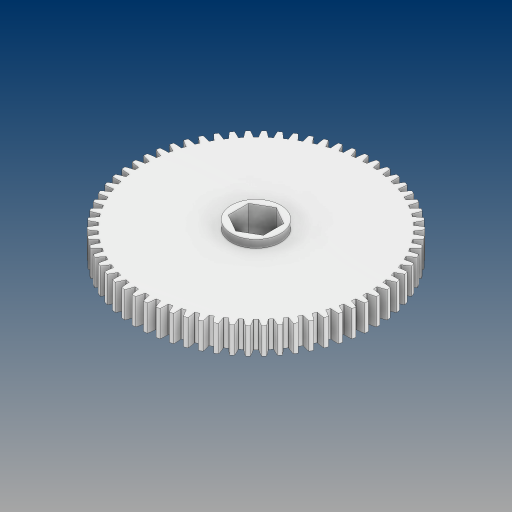
# Autodesk Inventor part: SHOT_1_004_66TGear-24TPulley
Saved by Autodesk Inventor 2024.3 (Build 283343000, 343)
## iProperties
Created: 2024-08-09
Part Number: SHOT_1_004_66TGear-24TPulley
Material: ABS Plastic
Document SubType Name: Modeling
Designer: Kenji
Density: 1.06 g/cm^3
Appearance: Smooth - White
Author: Kenji
Autodesk Inventor part; units mm, degrees
(part 1 of 3)
ref_plane "YZ Plane" through (0, 0, 0) normal (1, 0, 0) x (0, 1, 0)
ref_plane "XZ Plane" through (0, 0, 0) normal (0, 1, 0) x (-1, 0, 0)
ref_plane "XY Plane" through (0, 0, 0) normal (0, 0, 1) x (1, 0, 0)
sketch "Sketch1" plane through (0, 0, 0) normal (0, 1, 0) x (-1, 0, 0)
  circle A0 centre (0, 0) radius 41.91 construction
  line L0 (0, 0) -> (41.91, 0) construction
  line L1 (0, 0) -> (39.2827, 10.1592) construction
  line L2 (39.2827, 10.1592) -> (41.91, 0) construction
  arc A1 (39.2827, 10.1592) -> (37.9956, 14.2362) centre (0, 0) ccw construction
  arc A2 (40.5744, -0.225) -> (39.2827, 10.1592) centre (0, 0) ccw construction
  circle A3 centre (0, 0) radius 43.18
  line L3 (40.3225, 15.447) -> (40.3225, -15.447) construction
  line L4 (40.5744, -0.225) -> (41.91, 0) construction
  line L5 (40.5744, -0.225) -> (40.3225, -0.2901) construction
  line L6 (41.4814, 11.992) -> (38.8764, -18.7919) construction
  line L7 (40.5744, -0.225) -> (40.4457, -0.2469) construction
  line L8 (40.4457, -0.2469) -> (40.3225, -0.2901) construction
  line L9 (41.6879, 11.253) -> (38.5364, -19.4798) construction
  line L10 (40.5744, -0.225) -> (40.5099, -0.2348) construction
  line L11 (40.5099, -0.2348) -> (40.4457, -0.2469) construction
  line L12 (41.1912, 12.9537) -> (39.303, -17.8825) construction
  line L13 (40.5744, -0.225) -> (40.382, -0.2624) construction
  line L14 (40.4457, -0.2469) -> (40.382, -0.2624) construction
  line L15 (40.382, -0.2624) -> (40.3225, -0.2901) construction
  line L16 (37.9956, 14.2362) -> (43.1781, 0.4045) construction
  arc A4 (40.3121, -0.9596) -> (40.3225, -0.2901) centre (0, 0) ccw
  line L17 (40.3121, -0.9596) -> (0, 0) construction
  arc A5 (43.1678, -1.0276) -> (43.1781, 0.4045) centre (0, 0) ccw construction
  line L18 (43.1678, -1.0276) -> (40.3121, -0.9596) construction
  arc A6 (43.11, -2.4585) -> (43.1678, -1.0276) centre (0, 0) ccw construction
  arc A7 (40.2906, -1.6288) -> (40.3121, -0.9596) centre (0, 0) ccw
  line L19 (43.1781, 0.4045) -> (41.91, 0) construction
  line L20 (41.91, 0) -> (40.5744, -0.225) construction
  spline S0 degree 2 poles (43.1781, 0.4045) (41.91, 0) (40.5744, -0.225) knots 1 1 1 2 2 2
  line L21 (40.5744, -0.225) -> (40.5099, -0.2348) construction
  line L22 (40.5099, -0.2348) -> (40.4457, -0.2469) construction
  line L23 (40.4457, -0.2469) -> (40.382, -0.2624) construction
  line L24 (40.382, -0.2624) -> (40.3225, -0.2901) construction
  spline S1 degree 4 poles (40.5744, -0.225) (40.5099, -0.2348) (40.4457, -0.2469) (40.382, -0.2624) (40.3225, -0.2901) knots 1 1 1 1 1 2 2 2 2 2
  line L25 (43.11, -2.4585) -> (41.8625, -1.9942) construction
  line L26 (41.8625, -1.9942) -> (40.5392, -1.7059) construction
  spline S2 degree 2 poles (43.11, -2.4585) (41.8625, -1.9942) (40.5392, -1.7059) knots 1 1 1 2 2 2
  line L27 (40.5392, -1.7059) -> (40.4752, -1.693) construction
  line L28 (40.4752, -1.693) -> (40.4117, -1.6779) construction
  line L29 (40.4117, -1.6779) -> (40.3487, -1.6594) construction
  line L30 (40.3487, -1.6594) -> (40.2906, -1.6288) construction
  spline S3 degree 4 poles (40.5392, -1.7059) (40.4752, -1.693) (40.4117, -1.6779) (40.3487, -1.6594) (40.2906, -1.6288) knots 1 1 1 1 1 2 2 2 2 2
  line L31 (42.9441, 4.507) -> (41.7202, 3.9838) construction
  spline S4 degree 2 poles (42.9441, 4.507) (41.7202, 3.9838) (40.4121, 3.6329) knots 1 1 1 2 2 2
  line L32 (41.7202, 3.9838) -> (40.4121, 3.6329) construction
  spline S5 degree 2 poles (43.1484, 1.6505) (41.8625, 1.9942) (40.5178, 2.1553) knots 1 1 1 2 2 2
  line L33 (43.1484, 1.6505) -> (41.8625, 1.9942) construction
  line L34 (41.8625, 1.9942) -> (40.5178, 2.1553) construction
  line L35 (40.4528, 2.1621) -> (40.3882, 2.1711) construction
  spline S6 degree 4 poles (40.5178, 2.1553) (40.4528, 2.1621) (40.3882, 2.1711) (40.3237, 2.1835) (40.263, 2.2084) knots 1 1 1 1 1 2 2 2 2 2
  line L36 (40.5178, 2.1553) -> (40.4528, 2.1621) construction
  line L37 (40.3882, 2.1711) -> (40.3237, 2.1835) construction
  line L38 (40.3237, 2.1835) -> (40.263, 2.2084) construction
  arc A8 (40.263, 2.2084) -> (40.2208, 2.8766) centre (0, 0) ccw
  arc A9 (40.2208, 2.8766) -> (40.1675, 3.5441) centre (0, 0) ccw
  spline S7 degree 4 poles (40.4121, 3.6329) (40.3488, 3.617) (40.286, 3.5988) (40.224, 3.5774) (40.1675, 3.5441) knots 1 1 1 1 1 2 2 2 2 2
  line L39 (40.4121, 3.6329) -> (40.3488, 3.617) construction
  line L40 (40.3488, 3.617) -> (40.286, 3.5988) construction
  line L41 (40.286, 3.5988) -> (40.224, 3.5774) construction
  line L42 (40.224, 3.5774) -> (40.1675, 3.5441) construction
  line L43 (42.3213, 8.5687) -> (41.1526, 7.9315) construction
  spline S8 degree 2 poles (42.3213, 8.5687) (41.1526, 7.9315) (39.8838, 7.4578) knots 1 1 1 2 2 2
  line L44 (41.1526, 7.9315) -> (39.8838, 7.4578) construction
  spline S9 degree 2 poles (42.7962, 5.7445) (41.4834, 5.9644) (40.1294, 5.997) knots 1 1 1 2 2 2
  line L45 (42.7962, 5.7445) -> (41.4834, 5.9644) construction
  line L46 (41.4834, 5.9644) -> (40.1294, 5.997) construction
  line L47 (40.0641, 5.9976) -> (39.9989, 6.0004) construction
  spline S10 degree 4 poles (40.1294, 5.997) (40.0641, 5.9976) (39.9989, 6.0004) (39.9336, 6.0067) (39.8708, 6.0257) knots 1 1 1 1 1 2 2 2 2 2
  line L48 (40.1294, 5.997) -> (40.0641, 5.9976) construction
  line L49 (39.9989, 6.0004) -> (39.9336, 6.0067) construction
  line L50 (39.9336, 6.0067) -> (39.8708, 6.0257) construction
  arc A10 (39.8708, 6.0257) -> (39.7652, 6.6869) centre (0, 0) ccw
  arc A11 (39.7652, 6.6869) -> (39.6487, 7.3462) centre (0, 0) ccw
  spline S11 degree 4 poles (39.8838, 7.4578) (39.8223, 7.436) (39.7615, 7.412) (39.7019, 7.3847) (39.6487, 7.3462) knots 1 1 1 1 1 2 2 2 2 2
  line L51 (39.8838, 7.4578) -> (39.8223, 7.436) construction
  line L52 (39.8223, 7.436) -> (39.7615, 7.412) construction
  line L53 (39.7615, 7.412) -> (39.7019, 7.3847) construction
  line L54 (39.7019, 7.3847) -> (39.6487, 7.3462) construction
  line L55 (41.3151, 12.5528) -> (40.2124, 11.8074) construction
  spline S12 degree 2 poles (41.3151, 12.5528) (40.2124, 11.8074) (38.9943, 11.2153) knots 1 1 1 2 2 2
  line L56 (40.2124, 11.8074) -> (38.9943, 11.2153) construction
  spline S13 degree 2 poles (42.0563, 9.7866) (40.7286, 9.8807) (39.3777, 9.7844) knots 1 1 1 2 2 2
  line L57 (42.0563, 9.7866) -> (40.7286, 9.8807) construction
  line L58 (40.7286, 9.8807) -> (39.3777, 9.7844) construction
  line L59 (39.3126, 9.7787) -> (39.2474, 9.7754) construction
  spline S14 degree 4 poles (39.3777, 9.7844) (39.3126, 9.7787) (39.2474, 9.7754) (39.1818, 9.7754) (39.1175, 9.7883) knots 1 1 1 1 1 2 2 2 2 2
  line L60 (39.3777, 9.7844) -> (39.3126, 9.7787) construction
  line L61 (39.2474, 9.7754) -> (39.1818, 9.7754) construction
  line L62 (39.1818, 9.7754) -> (39.1175, 9.7883) construction
  arc A12 (39.1175, 9.7883) -> (38.9496, 10.4365) centre (0, 0) ccw
  arc A13 (38.9496, 10.4365) -> (38.7709, 11.0818) centre (0, 0) ccw
  spline S15 degree 4 poles (38.9943, 11.2153) (38.9351, 11.1877) (38.8769, 11.158) (38.8201, 11.1252) (38.7709, 11.0818) knots 1 1 1 1 1 2 2 2 2 2
  line L63 (38.9943, 11.2153) -> (38.9351, 11.1877) construction
  line L64 (38.9351, 11.1877) -> (38.8769, 11.158) construction
  line L65 (38.8769, 11.158) -> (38.8201, 11.1252) construction
  line L66 (38.8201, 11.1252) -> (38.7709, 11.0818) construction
  line L67 (39.9348, 16.4232) -> (38.9079, 15.5764) construction
  spline S16 degree 2 poles (39.9348, 16.4232) (38.9079, 15.5764) (37.7516, 14.8711) knots 1 1 1 2 2 2
  line L68 (38.9079, 15.5764) -> (37.7516, 14.8711) construction
  spline S17 degree 2 poles (40.9356, 13.7399) (39.605, 13.7074) (38.2693, 13.4832) knots 1 1 1 2 2 2
  line L69 (40.9356, 13.7399) -> (39.605, 13.7074) construction
  line L70 (39.605, 13.7074) -> (38.2693, 13.4832) construction
  line L71 (38.2051, 13.4714) -> (38.1405, 13.4618) construction
  spline S18 degree 4 poles (38.2693, 13.4832) (38.2051, 13.4714) (38.1405, 13.4618) (38.0752, 13.4556) (38.0099, 13.4624) knots 1 1 1 1 1 2 2 2 2 2
  line L72 (38.2693, 13.4832) -> (38.2051, 13.4714) construction
  line L73 (38.1405, 13.4618) -> (38.0752, 13.4556) construction
  line L74 (38.0752, 13.4556) -> (38.0099, 13.4624) construction
  arc A14 (38.0099, 13.4624) -> (37.7811, 14.0916) centre (0, 0) ccw
  arc A15 (37.7811, 14.0916) -> (37.5419, 14.717) centre (0, 0) ccw
  spline S19 degree 4 poles (37.7516, 14.8711) (37.6953, 14.838) (37.6403, 14.8029) (37.5868, 14.7649) (37.5419, 14.717) knots 1 1 1 1 1 2 2 2 2 2
  line L75 (37.7516, 14.8711) -> (37.6953, 14.838) construction
  line L76 (37.6953, 14.838) -> (37.6403, 14.8029) construction
  line L77 (37.6403, 14.8029) -> (37.5868, 14.7649) construction
  line L78 (37.5868, 14.7649) -> (37.5419, 14.717) construction
  line L79 (38.1929, 20.1449) -> (37.2511, 19.2043) construction
  spline S20 degree 2 poles (38.1929, 20.1449) (37.2511, 19.2043) (36.1671, 18.3923) knots 1 1 1 2 2 2
  line L80 (37.2511, 19.2043) -> (36.1671, 18.3923) construction
  spline S21 degree 2 poles (39.4442, 17.5689) (38.1227, 17.41) (36.8144, 17.0599) knots 1 1 1 2 2 2
  line L81 (39.4442, 17.5689) -> (38.1227, 17.41) construction
  line L82 (38.1227, 17.41) -> (36.8144, 17.0599) construction
  line L83 (36.7515, 17.042) -> (36.6882, 17.0263) construction
  spline S22 degree 4 poles (36.8144, 17.0599) (36.7515, 17.042) (36.6882, 17.0263) (36.6237, 17.0139) (36.5581, 17.0145) knots 1 1 1 1 1 2 2 2 2 2
  line L84 (36.8144, 17.0599) -> (36.7515, 17.042) construction
  line L85 (36.6882, 17.0263) -> (36.6237, 17.0139) construction
  line L86 (36.6237, 17.0139) -> (36.5581, 17.0145) construction
  arc A16 (36.5581, 17.0145) -> (36.2706, 17.6192) centre (0, 0) ccw
  arc A17 (36.2706, 17.6192) -> (35.973, 18.219) centre (0, 0) ccw
  spline S23 degree 4 poles (36.1671, 18.3923) (36.1142, 18.354) (36.0627, 18.3138) (36.0131, 18.2709) (35.973, 18.219) knots 1 1 1 1 1 2 2 2 2 2
  line L87 (36.1671, 18.3923) -> (36.1142, 18.354) construction
  line L88 (36.1142, 18.354) -> (36.0627, 18.3138) construction
  line L89 (36.0627, 18.3138) -> (36.0131, 18.2709) construction
  line L90 (36.0131, 18.2709) -> (35.973, 18.219) construction
  line L91 (36.1051, 23.6841) -> (35.2569, 22.6583) construction
  spline S24 degree 2 poles (36.1051, 23.6841) (35.2569, 22.6583) (34.255, 21.7469) knots 1 1 1 2 2 2
  line L92 (35.2569, 22.6583) -> (34.255, 21.7469) construction
  spline S25 degree 2 poles (37.5956, 21.2388) (36.2951, 20.955) (35.026, 20.4821) knots 1 1 1 2 2 2
  line L93 (37.5956, 21.2388) -> (36.2951, 20.955) construction
  line L94 (36.2951, 20.955) -> (35.026, 20.4821) construction
  line L95 (34.9652, 20.4583) -> (34.9036, 20.4367) construction
  spline S26 degree 4 poles (35.026, 20.4821) (34.9652, 20.4583) (34.9036, 20.4367) (34.8406, 20.4182) (34.7752, 20.4125) knots 1 1 1 1 1 2 2 2 2 2
  line L96 (35.026, 20.4821) -> (34.9652, 20.4583) construction
  line L97 (34.9036, 20.4367) -> (34.8406, 20.4182) construction
  line L98 (34.8406, 20.4182) -> (34.7752, 20.4125) construction
  arc A18 (34.7752, 20.4125) -> (34.4315, 20.9871) centre (0, 0) ccw
  arc A19 (34.4315, 20.9871) -> (34.0783, 21.5559) centre (0, 0) ccw
  spline S27 degree 4 poles (34.255, 21.7469) (34.206, 21.7038) (34.1586, 21.6589) (34.1133, 21.6114) (34.0783, 21.5559) knots 1 1 1 1 1 2 2 2 2 2
  line L99 (34.255, 21.7469) -> (34.206, 21.7038) construction
  line L100 (34.206, 21.7038) -> (34.1586, 21.6589) construction
  line L101 (34.1586, 21.6589) -> (34.1133, 21.6114) construction
  line L102 (34.1133, 21.6114) -> (34.0783, 21.5559) construction
  line L103 (33.6903, 27.0089) -> (32.9435, 25.907) construction
  spline S28 degree 2 poles (33.6903, 27.0089) (32.9435, 25.907) (32.0327, 24.9046) knots 1 1 1 2 2 2
  line L104 (32.9435, 25.907) -> (32.0327, 24.9046) construction
  spline S29 degree 2 poles (35.4065, 24.7163) (34.1389, 24.3102) (32.9205, 23.7188) knots 1 1 1 2 2 2
  line L105 (35.4065, 24.7163) -> (34.1389, 24.3102) construction
  line L106 (34.1389, 24.3102) -> (32.9205, 23.7188) construction
  line L107 (32.8622, 23.6893) -> (32.8029, 23.6619) construction
  spline S30 degree 4 poles (32.9205, 23.7188) (32.8622, 23.6893) (32.8029, 23.6619) (32.742, 23.6376) (32.6774, 23.6257) knots 1 1 1 1 1 2 2 2 2 2
  line L108 (32.9205, 23.7188) -> (32.8622, 23.6893) construction
  line L109 (32.8029, 23.6619) -> (32.742, 23.6376) construction
  line L110 (32.742, 23.6376) -> (32.6774, 23.6257) construction
  arc A20 (32.6774, 23.6257) -> (32.2807, 24.165) centre (0, 0) ccw
  arc A21 (32.2807, 24.165) -> (31.875, 24.6977) centre (0, 0) ccw
  spline S31 degree 4 poles (32.0327, 24.9046) (31.9881, 24.857) (31.9451, 24.8078) (31.9046, 24.7562) (31.875, 24.6977) knots 1 1 1 1 1 2 2 2 2 2
  line L111 (32.0327, 24.9046) -> (31.9881, 24.857) construction
  line L112 (31.9881, 24.857) -> (31.9451, 24.8078) construction
  line L113 (31.9451, 24.8078) -> (31.9046, 24.7562) construction
  line L114 (31.9046, 24.7562) -> (31.875, 24.6977) construction
  line L115 (30.9703, 30.089) -> (30.3317, 28.9212) construction
  spline S32 degree 2 poles (30.9703, 30.089) (30.3317, 28.9212) (29.5204, 27.8367) knots 1 1 1 2 2 2
  line L116 (30.3317, 28.9212) -> (29.5204, 27.8367) construction
  spline S33 degree 2 poles (32.8967, 27.97) (31.6735, 27.4452) (30.5168, 26.7406) knots 1 1 1 2 2 2
  line L117 (32.8967, 27.97) -> (31.6735, 27.4452) construction
  line L118 (31.6735, 27.4452) -> (30.5168, 26.7406) construction
  line L119 (30.4616, 26.7058) -> (30.4051, 26.6729) construction
  spline S34 degree 4 poles (30.5168, 26.7406) (30.4616, 26.7058) (30.4051, 26.6729) (30.3468, 26.6429) (30.2837, 26.6249) knots 1 1 1 1 1 2 2 2 2 2
  line L120 (30.5168, 26.7406) -> (30.4616, 26.7058) construction
  line L121 (30.4051, 26.6729) -> (30.3468, 26.6429) construction
  line L122 (30.3468, 26.6429) -> (30.2837, 26.6249) construction
  arc A22 (30.2837, 26.6249) -> (29.8375, 27.1241) centre (0, 0) ccw
  arc A23 (29.8375, 27.1241) -> (29.383, 27.6157) centre (0, 0) ccw
  spline S35 degree 4 poles (29.5204, 27.8367) (29.4804, 27.7851) (29.4423, 27.732) (29.4069, 27.6768) (29.383, 27.6157) knots 1 1 1 1 1 2 2 2 2 2
  line L123 (29.5204, 27.8367) -> (29.4804, 27.7851) construction
  line L124 (29.4804, 27.7851) -> (29.4423, 27.732) construction
  line L125 (29.4423, 27.732) -> (29.4069, 27.6768) construction
  line L126 (29.4069, 27.6768) -> (29.383, 27.6157) construction
  line L127 (27.97, 32.8967) -> (27.4452, 31.6735) construction
  spline S36 degree 2 poles (27.97, 32.8967) (27.4452, 31.6735) (26.7406, 30.5168) knots 1 1 1 2 2 2
  line L128 (27.4452, 31.6735) -> (26.7406, 30.5168) construction
  spline S37 degree 2 poles (30.089, 30.9703) (28.9212, 30.3317) (27.8367, 29.5204) knots 1 1 1 2 2 2
  line L129 (30.089, 30.9703) -> (28.9212, 30.3317) construction
  line L130 (28.9212, 30.3317) -> (27.8367, 29.5204) construction
  line L131 (27.7851, 29.4804) -> (27.732, 29.4423) construction
  spline S38 degree 4 poles (27.8367, 29.5204) (27.7851, 29.4804) (27.732, 29.4423) (27.6768, 29.4069) (27.6157, 29.383) knots 1 1 1 1 1 2 2 2 2 2
  line L132 (27.8367, 29.5204) -> (27.7851, 29.4804) construction
  line L133 (27.732, 29.4423) -> (27.6768, 29.4069) construction
  line L134 (27.6768, 29.4069) -> (27.6157, 29.383) construction
  arc A24 (27.6157, 29.383) -> (27.1241, 29.8375) centre (0, 0) ccw
  arc A25 (27.1241, 29.8375) -> (26.6249, 30.2837) centre (0, 0) ccw
  spline S39 degree 4 poles (26.7406, 30.5168) (26.7058, 30.4616) (26.6729, 30.4051) (26.6429, 30.3468) (26.6249, 30.2837) knots 1 1 1 1 1 2 2 2 2 2
  line L135 (26.7406, 30.5168) -> (26.7058, 30.4616) construction
  line L136 (26.7058, 30.4616) -> (26.6729, 30.4051) construction
  line L137 (26.6729, 30.4051) -> (26.6429, 30.3468) construction
  line L138 (26.6429, 30.3468) -> (26.6249, 30.2837) construction
  line L139 (24.7163, 35.4065) -> (24.3102, 34.1389) construction
  spline S40 degree 2 poles (24.7163, 35.4065) (24.3102, 34.1389) (23.7188, 32.9205) knots 1 1 1 2 2 2
  line L140 (24.3102, 34.1389) -> (23.7188, 32.9205) construction
  spline S41 degree 2 poles (27.0089, 33.6903) (25.907, 32.9435) (24.9046, 32.0327) knots 1 1 1 2 2 2
  line L141 (27.0089, 33.6903) -> (25.907, 32.9435) construction
  line L142 (25.907, 32.9435) -> (24.9046, 32.0327) construction
  line L143 (24.857, 31.9881) -> (24.8078, 31.9451) construction
  spline S42 degree 4 poles (24.9046, 32.0327) (24.857, 31.9881) (24.8078, 31.9451) (24.7562, 31.9046) (24.6977, 31.875) knots 1 1 1 1 1 2 2 2 2 2
  line L144 (24.9046, 32.0327) -> (24.857, 31.9881) construction
  line L145 (24.8078, 31.9451) -> (24.7562, 31.9046) construction
  line L146 (24.7562, 31.9046) -> (24.6977, 31.875) construction
  arc A26 (24.6977, 31.875) -> (24.165, 32.2807) centre (0, 0) ccw
  arc A27 (24.165, 32.2807) -> (23.6257, 32.6774) centre (0, 0) ccw
  spline S43 degree 4 poles (23.7188, 32.9205) (23.6893, 32.8622) (23.6619, 32.8029) (23.6376, 32.742) (23.6257, 32.6774) knots 1 1 1 1 1 2 2 2 2 2
  line L147 (23.7188, 32.9205) -> (23.6893, 32.8622) construction
  line L148 (23.6893, 32.8622) -> (23.6619, 32.8029) construction
  line L149 (23.6619, 32.8029) -> (23.6376, 32.742) construction
  line L150 (23.6376, 32.742) -> (23.6257, 32.6774) construction
  line L151 (21.2388, 37.5956) -> (20.955, 36.2951) construction
  spline S44 degree 2 poles (21.2388, 37.5956) (20.955, 36.2951) (20.4821, 35.026) knots 1 1 1 2 2 2
  line L152 (20.955, 36.2951) -> (20.4821, 35.026) construction
  spline S45 degree 2 poles (23.6841, 36.1051) (22.6583, 35.2569) (21.7469, 34.255) knots 1 1 1 2 2 2
  line L153 (23.6841, 36.1051) -> (22.6583, 35.2569) construction
  line L154 (22.6583, 35.2569) -> (21.7469, 34.255) construction
  line L155 (21.7038, 34.206) -> (21.6589, 34.1586) construction
  spline S46 degree 4 poles (21.7469, 34.255) (21.7038, 34.206) (21.6589, 34.1586) (21.6114, 34.1133) (21.5559, 34.0783) knots 1 1 1 1 1 2 2 2 2 2
  line L156 (21.7469, 34.255) -> (21.7038, 34.206) construction
  line L157 (21.6589, 34.1586) -> (21.6114, 34.1133) construction
  line L158 (21.6114, 34.1133) -> (21.5559, 34.0783) construction
  arc A28 (21.5559, 34.0783) -> (20.9871, 34.4315) centre (0, 0) ccw
  arc A29 (20.9871, 34.4315) -> (20.4125, 34.7752) centre (0, 0) ccw
  spline S47 degree 4 poles (20.4821, 35.026) (20.4583, 34.9652) (20.4367, 34.9036) (20.4182, 34.8406) (20.4125, 34.7752) knots 1 1 1 1 1 2 2 2 2 2
  line L159 (20.4821, 35.026) -> (20.4583, 34.9652) construction
  line L160 (20.4583, 34.9652) -> (20.4367, 34.9036) construction
  line L161 (20.4367, 34.9036) -> (20.4182, 34.8406) construction
  line L162 (20.4182, 34.8406) -> (20.4125, 34.7752) construction
  line L163 (17.5689, 39.4442) -> (17.41, 38.1227) construction
  spline S48 degree 2 poles (17.5689, 39.4442) (17.41, 38.1227) (17.0599, 36.8144) knots 1 1 1 2 2 2
  line L164 (17.41, 38.1227) -> (17.0599, 36.8144) construction
  spline S49 degree 2 poles (20.1449, 38.1929) (19.2043, 37.2511) (18.3923, 36.1671) knots 1 1 1 2 2 2
  line L165 (20.1449, 38.1929) -> (19.2043, 37.2511) construction
  line L166 (19.2043, 37.2511) -> (18.3923, 36.1671) construction
  line L167 (18.354, 36.1142) -> (18.3138, 36.0627) construction
  spline S50 degree 4 poles (18.3923, 36.1671) (18.354, 36.1142) (18.3138, 36.0627) (18.2709, 36.0131) (18.219, 35.973) knots 1 1 1 1 1 2 2 2 2 2
  line L168 (18.3923, 36.1671) -> (18.354, 36.1142) construction
  line L169 (18.3138, 36.0627) -> (18.2709, 36.0131) construction
  line L170 (18.2709, 36.0131) -> (18.219, 35.973) construction
  arc A30 (18.219, 35.973) -> (17.6192, 36.2706) centre (0, 0) ccw
  arc A31 (17.6192, 36.2706) -> (17.0145, 36.5581) centre (0, 0) ccw
  spline S51 degree 4 poles (17.0599, 36.8144) (17.042, 36.7515) (17.0263, 36.6882) (17.0139, 36.6237) (17.0145, 36.5581) knots 1 1 1 1 1 2 2 2 2 2
  line L171 (17.0599, 36.8144) -> (17.042, 36.7515) construction
  line L172 (17.042, 36.7515) -> (17.0263, 36.6882) construction
  line L173 (17.0263, 36.6882) -> (17.0139, 36.6237) construction
  line L174 (17.0139, 36.6237) -> (17.0145, 36.5581) construction
  line L175 (13.7399, 40.9356) -> (13.7074, 39.605) construction
  spline S52 degree 2 poles (13.7399, 40.9356) (13.7074, 39.605) (13.4832, 38.2693) knots 1 1 1 2 2 2
  line L176 (13.7074, 39.605) -> (13.4832, 38.2693) construction
  spline S53 degree 2 poles (16.4232, 39.9348) (15.5764, 38.9079) (14.8711, 37.7516) knots 1 1 1 2 2 2
  line L177 (16.4232, 39.9348) -> (15.5764, 38.9079) construction
  line L178 (15.5764, 38.9079) -> (14.8711, 37.7516) construction
  line L179 (14.838, 37.6953) -> (14.8029, 37.6403) construction
  spline S54 degree 4 poles (14.8711, 37.7516) (14.838, 37.6953) (14.8029, 37.6403) (14.7649, 37.5868) (14.717, 37.5419) knots 1 1 1 1 1 2 2 2 2 2
  line L180 (14.8711, 37.7516) -> (14.838, 37.6953) construction
  line L181 (14.8029, 37.6403) -> (14.7649, 37.5868) construction
  line L182 (14.7649, 37.5868) -> (14.717, 37.5419) construction
  arc A32 (14.717, 37.5419) -> (14.0916, 37.7811) centre (0, 0) ccw
  arc A33 (14.0916, 37.7811) -> (13.4624, 38.0099) centre (0, 0) ccw
  spline S55 degree 4 poles (13.4832, 38.2693) (13.4714, 38.2051) (13.4618, 38.1405) (13.4556, 38.0752) (13.4624, 38.0099) knots 1 1 1 1 1 2 2 2 2 2
  line L183 (13.4832, 38.2693) -> (13.4714, 38.2051) construction
  line L184 (13.4714, 38.2051) -> (13.4618, 38.1405) construction
  line L185 (13.4618, 38.1405) -> (13.4556, 38.0752) construction
  line L186 (13.4556, 38.0752) -> (13.4624, 38.0099) construction
  line L187 (9.7866, 42.0563) -> (9.8807, 40.7286) construction
  spline S56 degree 2 poles (9.7866, 42.0563) (9.8807, 40.7286) (9.7844, 39.3777) knots 1 1 1 2 2 2
  line L188 (9.8807, 40.7286) -> (9.7844, 39.3777) construction
  spline S57 degree 2 poles (12.5528, 41.3151) (11.8074, 40.2124) (11.2153, 38.9943) knots 1 1 1 2 2 2
  line L189 (12.5528, 41.3151) -> (11.8074, 40.2124) construction
  line L190 (11.8074, 40.2124) -> (11.2153, 38.9943) construction
  line L191 (11.1877, 38.9351) -> (11.158, 38.8769) construction
  spline S58 degree 4 poles (11.2153, 38.9943) (11.1877, 38.9351) (11.158, 38.8769) (11.1252, 38.8201) (11.0818, 38.7709) knots 1 1 1 1 1 2 2 2 2 2
  line L192 (11.2153, 38.9943) -> (11.1877, 38.9351) construction
  line L193 (11.158, 38.8769) -> (11.1252, 38.8201) construction
  line L194 (11.1252, 38.8201) -> (11.0818, 38.7709) construction
  arc A34 (11.0818, 38.7709) -> (10.4365, 38.9496) centre (0, 0) ccw
  arc A35 (10.4365, 38.9496) -> (9.7883, 39.1175) centre (0, 0) ccw
  spline S59 degree 4 poles (9.7844, 39.3777) (9.7787, 39.3126) (9.7754, 39.2474) (9.7754, 39.1818) (9.7883, 39.1175) knots 1 1 1 1 1 2 2 2 2 2
  line L195 (9.7844, 39.3777) -> (9.7787, 39.3126) construction
  line L196 (9.7787, 39.3126) -> (9.7754, 39.2474) construction
  line L197 (9.7754, 39.2474) -> (9.7754, 39.1818) construction
  line L198 (9.7754, 39.1818) -> (9.7883, 39.1175) construction
  line L199 (5.7445, 42.7962) -> (5.9644, 41.4834) construction
  spline S60 degree 2 poles (5.7445, 42.7962) (5.9644, 41.4834) (5.997, 40.1294) knots 1 1 1 2 2 2
  line L200 (5.9644, 41.4834) -> (5.997, 40.1294) construction
  spline S61 degree 2 poles (8.5687, 42.3213) (7.9315, 41.1526) (7.4578, 39.8838) knots 1 1 1 2 2 2
  line L201 (8.5687, 42.3213) -> (7.9315, 41.1526) construction
  line L202 (7.9315, 41.1526) -> (7.4578, 39.8838) construction
  line L203 (7.436, 39.8223) -> (7.412, 39.7615) construction
  spline S62 degree 4 poles (7.4578, 39.8838) (7.436, 39.8223) (7.412, 39.7615) (7.3847, 39.7019) (7.3462, 39.6487) knots 1 1 1 1 1 2 2 2 2 2
  line L204 (7.4578, 39.8838) -> (7.436, 39.8223) construction
  line L205 (7.412, 39.7615) -> (7.3847, 39.7019) construction
  line L206 (7.3847, 39.7019) -> (7.3462, 39.6487) construction
  arc A36 (7.3462, 39.6487) -> (6.6869, 39.7652) centre (0, 0) ccw
  arc A37 (6.6869, 39.7652) -> (6.0257, 39.8708) centre (0, 0) ccw
  spline S63 degree 4 poles (5.997, 40.1294) (5.9976, 40.0641) (6.0004, 39.9989) (6.0067, 39.9336) (6.0257, 39.8708) knots 1 1 1 1 1 2 2 2 2 2
  line L207 (5.997, 40.1294) -> (5.9976, 40.0641) construction
  line L208 (5.9976, 40.0641) -> (6.0004, 39.9989) construction
  line L209 (6.0004, 39.9989) -> (6.0067, 39.9336) construction
  line L210 (6.0067, 39.9336) -> (6.0257, 39.8708) construction
  line L211 (1.6505, 43.1484) -> (1.9942, 41.8625) construction
  spline S64 degree 2 poles (1.6505, 43.1484) (1.9942, 41.8625) (2.1553, 40.5178) knots 1 1 1 2 2 2
  line L212 (1.9942, 41.8625) -> (2.1553, 40.5178) construction
  spline S65 degree 2 poles (4.507, 42.9441) (3.9838, 41.7202) (3.6329, 40.4121) knots 1 1 1 2 2 2
  line L213 (4.507, 42.9441) -> (3.9838, 41.7202) construction
  line L214 (3.9838, 41.7202) -> (3.6329, 40.4121) construction
  line L215 (3.617, 40.3488) -> (3.5988, 40.286) construction
  spline S66 degree 4 poles (3.6329, 40.4121) (3.617, 40.3488) (3.5988, 40.286) (3.5774, 40.224) (3.5441, 40.1675) knots 1 1 1 1 1 2 2 2 2 2
  line L216 (3.6329, 40.4121) -> (3.617, 40.3488) construction
  line L217 (3.5988, 40.286) -> (3.5774, 40.224) construction
  line L218 (3.5774, 40.224) -> (3.5441, 40.1675) construction
  arc A38 (3.5441, 40.1675) -> (2.8766, 40.2208) centre (0, 0) ccw
  arc A39 (2.8766, 40.2208) -> (2.2084, 40.263) centre (0, 0) ccw
  spline S67 degree 4 poles (2.1553, 40.5178) (2.1621, 40.4528) (2.1711, 40.3882) (2.1835, 40.3237) (2.2084, 40.263) knots 1 1 1 1 1 2 2 2 2 2
  line L219 (2.1553, 40.5178) -> (2.1621, 40.4528) construction
  line L220 (2.1621, 40.4528) -> (2.1711, 40.3882) construction
  line L221 (2.1711, 40.3882) -> (2.1835, 40.3237) construction
  line L222 (2.1835, 40.3237) -> (2.2084, 40.263) construction
  line L223 (-2.4585, 43.11) -> (-1.9942, 41.8625) construction
  spline S68 degree 2 poles (-2.4585, 43.11) (-1.9942, 41.8625) (-1.7059, 40.5392) knots 1 1 1 2 2 2
  line L224 (-1.9942, 41.8625) -> (-1.7059, 40.5392) construction
  spline S69 degree 2 poles (0.4045, 43.1781) (0, 41.91) (-0.225, 40.5744) knots 1 1 1 2 2 2
  line L225 (0.4045, 43.1781) -> (0, 41.91) construction
  line L226 (0, 41.91) -> (-0.225, 40.5744) construction
  line L227 (-0.2348, 40.5099) -> (-0.2469, 40.4457) construction
  spline S70 degree 4 poles (-0.225, 40.5744) (-0.2348, 40.5099) (-0.2469, 40.4457) (-0.2624, 40.382) (-0.2901, 40.3225) knots 1 1 1 1 1 2 2 2 2 2
  line L228 (-0.225, 40.5744) -> (-0.2348, 40.5099) construction
  line L229 (-0.2469, 40.4457) -> (-0.2624, 40.382) construction
  line L230 (-0.2624, 40.382) -> (-0.2901, 40.3225) construction
  arc A40 (-0.2901, 40.3225) -> (-0.9596, 40.3121) centre (0, 0) ccw
  arc A41 (-0.9596, 40.3121) -> (-1.6288, 40.2906) centre (0, 0) ccw
  spline S71 degree 4 poles (-1.7059, 40.5392) (-1.693, 40.4752) (-1.6779, 40.4117) (-1.6594, 40.3487) (-1.6288, 40.2906) knots 1 1 1 1 1 2 2 2 2 2
  line L231 (-1.7059, 40.5392) -> (-1.693, 40.4752) construction
  line L232 (-1.693, 40.4752) -> (-1.6779, 40.4117) construction
  line L233 (-1.6779, 40.4117) -> (-1.6594, 40.3487) construction
  line L234 (-1.6594, 40.3487) -> (-1.6288, 40.2906) construction
  line L235 (-6.5452, 42.6811) -> (-5.9644, 41.4834) construction
  spline S72 degree 2 poles (-6.5452, 42.6811) (-5.9644, 41.4834) (-5.5517, 40.1935) knots 1 1 1 2 2 2
  line L236 (-5.9644, 41.4834) -> (-5.5517, 40.1935) construction
  spline S73 degree 2 poles (-3.7017, 43.021) (-3.9838, 41.7202) (-4.0808, 40.3693) knots 1 1 1 2 2 2
  line L237 (-3.7017, 43.021) -> (-3.9838, 41.7202) construction
  line L238 (-3.9838, 41.7202) -> (-4.0808, 40.3693) construction
  line L239 (-4.0844, 40.3041) -> (-4.0904, 40.2391) construction
  spline S74 degree 4 poles (-4.0808, 40.3693) (-4.0844, 40.3041) (-4.0904, 40.2391) (-4.0997, 40.1742) (-4.1217, 40.1123) knots 1 1 1 1 1 2 2 2 2 2
  line L240 (-4.0808, 40.3693) -> (-4.0844, 40.3041) construction
  line L241 (-4.0904, 40.2391) -> (-4.0997, 40.1742) construction
  line L242 (-4.0997, 40.1742) -> (-4.1217, 40.1123) construction
  arc A42 (-4.1217, 40.1123) -> (-4.7872, 40.0384) centre (0, 0) ccw
  arc A43 (-4.7872, 40.0384) -> (-5.4513, 39.9534) centre (0, 0) ccw
  spline S75 degree 4 poles (-5.5517, 40.1935) (-5.5328, 40.131) (-5.5116, 40.0692) (-5.4872, 40.0083) (-5.4513, 39.9534) knots 1 1 1 1 1 2 2 2 2 2
  line L243 (-5.5517, 40.1935) -> (-5.5328, 40.131) construction
  line L244 (-5.5328, 40.131) -> (-5.5116, 40.0692) construction
  line L245 (-5.5116, 40.0692) -> (-5.4872, 40.0083) construction
  line L246 (-5.4872, 40.0083) -> (-5.4513, 39.9534) construction
  line L247 (-10.5727, 41.8656) -> (-9.8807, 40.7286) construction
  spline S76 degree 2 poles (-10.5727, 41.8656) (-9.8807, 40.7286) (-9.3471, 39.4838) knots 1 1 1 2 2 2
  line L248 (-9.8807, 40.7286) -> (-9.3471, 39.4838) construction
  spline S77 degree 2 poles (-7.7743, 42.4744) (-7.9315, 41.1526) (-7.8997, 39.7986) knots 1 1 1 2 2 2
  line L249 (-7.7743, 42.4744) -> (-7.9315, 41.1526) construction
  line L250 (-7.9315, 41.1526) -> (-7.8997, 39.7986) construction
  line L251 (-7.8971, 39.7334) -> (-7.8968, 39.6681) construction
  spline S78 degree 4 poles (-7.8997, 39.7986) (-7.8971, 39.7334) (-7.8968, 39.6681) (-7.9, 39.6025) (-7.916, 39.5389) knots 1 1 1 1 1 2 2 2 2 2
  line L252 (-7.8997, 39.7986) -> (-7.8971, 39.7334) construction
  line L253 (-7.8968, 39.6681) -> (-7.9, 39.6025) construction
  line L254 (-7.9, 39.6025) -> (-7.916, 39.5389) construction
  arc A44 (-7.916, 39.5389) -> (-8.5714, 39.402) centre (0, 0) ccw
  arc A45 (-8.5714, 39.402) -> (-9.2244, 39.2543) centre (0, 0) ccw
  spline S79 degree 4 poles (-9.3471, 39.4838) (-9.3224, 39.4233) (-9.2955, 39.3638) (-9.2654, 39.3055) (-9.2244, 39.2543) knots 1 1 1 1 1 2 2 2 2 2
  line L255 (-9.3471, 39.4838) -> (-9.3224, 39.4233) construction
  line L256 (-9.3224, 39.4233) -> (-9.2955, 39.3638) construction
  line L257 (-9.2955, 39.3638) -> (-9.2654, 39.3055) construction
  line L258 (-9.2654, 39.3055) -> (-9.2244, 39.2543) construction
  line L259 (-14.5044, 40.6711) -> (-13.7074, 39.605) construction
  spline S80 degree 2 poles (-14.5044, 40.6711) (-13.7074, 39.605) (-13.058, 38.4165) knots 1 1 1 2 2 2
  line L260 (-13.7074, 39.605) -> (-13.058, 38.4165) construction
  spline S81 degree 2 poles (-11.7766, 41.543) (-11.8074, 40.2124) (-11.647, 38.8675) knots 1 1 1 2 2 2
  line L261 (-11.7766, 41.543) -> (-11.8074, 40.2124) construction
  line L262 (-11.8074, 40.2124) -> (-11.647, 38.8675) construction
  line L263 (-11.6382, 38.8028) -> (-11.6318, 38.7378) construction
  spline S82 degree 4 poles (-11.647, 38.8675) (-11.6382, 38.8028) (-11.6318, 38.7378) (-11.6287, 38.6723) (-11.6385, 38.6074) knots 1 1 1 1 1 2 2 2 2 2
  line L264 (-11.647, 38.8675) -> (-11.6382, 38.8028) construction
  line L265 (-11.6318, 38.7378) -> (-11.6287, 38.6723) construction
  line L266 (-11.6287, 38.6723) -> (-11.6385, 38.6074) construction
  arc A46 (-11.6385, 38.6074) -> (-12.278, 38.4088) centre (0, 0) ccw
  arc A47 (-12.278, 38.4088) -> (-12.914, 38.1997) centre (0, 0) ccw
  spline S83 degree 4 poles (-13.058, 38.4165) (-13.0276, 38.3587) (-12.9952, 38.302) (-12.9597, 38.2468) (-12.914, 38.1997) knots 1 1 1 1 1 2 2 2 2 2
  line L267 (-13.058, 38.4165) -> (-13.0276, 38.3587) construction
  line L268 (-13.0276, 38.3587) -> (-12.9952, 38.302) construction
  line L269 (-12.9952, 38.302) -> (-12.9597, 38.2468) construction
  line L270 (-12.9597, 38.2468) -> (-12.914, 38.1997) construction
  line L271 (-18.3048, 39.1082) -> (-17.41, 38.1227) construction
  spline S84 degree 2 poles (-18.3048, 39.1082) (-17.41, 38.1227) (-16.6506, 37.0013) knots 1 1 1 2 2 2
  line L272 (-17.41, 38.1227) -> (-16.6506, 37.0013) construction
  spline S85 degree 2 poles (-15.6722, 40.2355) (-15.5764, 38.9079) (-15.2889, 37.5844) knots 1 1 1 2 2 2
  line L273 (-15.6722, 40.2355) -> (-15.5764, 38.9079) construction
  line L274 (-15.5764, 38.9079) -> (-15.2889, 37.5844) construction
  line L275 (-15.274, 37.5208) -> (-15.2614, 37.4567) construction
  spline S86 degree 4 poles (-15.2889, 37.5844) (-15.274, 37.5208) (-15.2614, 37.4567) (-15.252, 37.3918) (-15.2557, 37.3263) knots 1 1 1 1 1 2 2 2 2 2
  line L276 (-15.2889, 37.5844) -> (-15.274, 37.5208) construction
  line L277 (-15.2614, 37.4567) -> (-15.252, 37.3918) construction
  line L278 (-15.252, 37.3918) -> (-15.2557, 37.3263) construction
  arc A48 (-15.2557, 37.3263) -> (-15.8734, 37.0678) centre (0, 0) ccw
  arc A49 (-15.8734, 37.0678) -> (-16.4867, 36.7992) centre (0, 0) ccw
  spline S87 degree 4 poles (-16.6506, 37.0013) (-16.6148, 36.9466) (-16.5772, 36.8933) (-16.5366, 36.8417) (-16.4867, 36.7992) knots 1 1 1 1 1 2 2 2 2 2
  line L279 (-16.6506, 37.0013) -> (-16.6148, 36.9466) construction
  line L280 (-16.6148, 36.9466) -> (-16.5772, 36.8933) construction
  line L281 (-16.5772, 36.8933) -> (-16.5366, 36.8417) construction
  line L282 (-16.5366, 36.8417) -> (-16.4867, 36.7992) construction
  line L283 (-21.9393, 37.1911) -> (-20.955, 36.2951) construction
  spline S88 degree 2 poles (-21.9393, 37.1911) (-20.955, 36.2951) (-20.0924, 35.251) knots 1 1 1 2 2 2
  line L284 (-20.955, 36.2951) -> (-20.0924, 35.251) construction
  spline S89 degree 2 poles (-19.4258, 38.5636) (-19.2043, 37.2511) (-18.7923, 35.9609) knots 1 1 1 2 2 2
  line L285 (-19.4258, 38.5636) -> (-19.2043, 37.2511) construction
  line L286 (-19.2043, 37.2511) -> (-18.7923, 35.9609) construction
  line L287 (-18.7714, 35.899) -> (-18.7528, 35.8364) construction
  spline S90 degree 4 poles (-18.7923, 35.9609) (-18.7714, 35.899) (-18.7528, 35.8364) (-18.7373, 35.7727) (-18.7347, 35.7071) knots 1 1 1 1 1 2 2 2 2 2
  line L288 (-18.7923, 35.9609) -> (-18.7714, 35.899) construction
  line L289 (-18.7528, 35.8364) -> (-18.7373, 35.7727) construction
  line L290 (-18.7373, 35.7727) -> (-18.7347, 35.7071) construction
  arc A50 (-18.7347, 35.7071) -> (-19.325, 35.3911) centre (0, 0) ccw
  arc A51 (-19.325, 35.3911) -> (-19.91, 35.0654) centre (0, 0) ccw
  spline S91 degree 4 poles (-20.0924, 35.251) (-20.0516, 35.2) (-20.009, 35.1505) (-19.9637, 35.103) (-19.91, 35.0654) knots 1 1 1 1 1 2 2 2 2 2
  line L291 (-20.0924, 35.251) -> (-20.0516, 35.2) construction
  line L292 (-20.0516, 35.2) -> (-20.009, 35.1505) construction
  line L293 (-20.009, 35.1505) -> (-19.9637, 35.103) construction
  line L294 (-19.9637, 35.103) -> (-19.91, 35.0654) construction
  line L295 (-25.3752, 34.9372) -> (-24.3102, 34.1389) construction
  spline S92 degree 2 poles (-25.3752, 34.9372) (-24.3102, 34.1389) (-23.3522, 33.1815) knots 1 1 1 2 2 2
  line L296 (-24.3102, 34.1389) -> (-23.3522, 33.1815) construction
  spline S93 degree 2 poles (-23.0036, 36.5424) (-22.6583, 35.2569) (-22.1255, 34.0118) knots 1 1 1 2 2 2
  line L297 (-23.0036, 36.5424) -> (-22.6583, 35.2569) construction
  line L298 (-22.6583, 35.2569) -> (-22.1255, 34.0118) construction
  line L299 (-22.0988, 33.9521) -> (-22.0743, 33.8916) construction
  spline S94 degree 4 poles (-22.1255, 34.0118) (-22.0988, 33.9521) (-22.0743, 33.8916) (-22.0529, 33.8296) (-22.0441, 33.7646) knots 1 1 1 1 1 2 2 2 2 2
  line L300 (-22.1255, 34.0118) -> (-22.0988, 33.9521) construction
  line L301 (-22.0743, 33.8916) -> (-22.0529, 33.8296) construction
  line L302 (-22.0529, 33.8296) -> (-22.0441, 33.7646) construction
  arc A52 (-22.0441, 33.7646) -> (-22.6017, 33.3939) centre (0, 0) ccw
  arc A53 (-22.6017, 33.3939) -> (-23.153, 33.014) centre (0, 0) ccw
  spline S95 degree 4 poles (-23.3522, 33.1815) (-23.3068, 33.1346) (-23.2597, 33.0893) (-23.2101, 33.0464) (-23.153, 33.014) knots 1 1 1 1 1 2 2 2 2 2
  line L303 (-23.3522, 33.1815) -> (-23.3068, 33.1346) construction
  line L304 (-23.3068, 33.1346) -> (-23.2597, 33.0893) construction
  line L305 (-23.2597, 33.0893) -> (-23.2101, 33.0464) construction
  line L306 (-23.2101, 33.0464) -> (-23.153, 33.014) construction
  line L307 (-28.5813, 32.367) -> (-27.4452, 31.6735) construction
  spline S96 degree 2 poles (-28.5813, 32.367) (-27.4452, 31.6735) (-26.4006, 30.8115) knots 1 1 1 2 2 2
  line L308 (-27.4452, 31.6735) -> (-26.4006, 30.8115) construction
  spline S97 degree 2 poles (-26.373, 34.1903) (-25.907, 32.9435) (-25.2583, 31.7546) knots 1 1 1 2 2 2
  line L309 (-26.373, 34.1903) -> (-25.907, 32.9435) construction
  line L310 (-25.907, 32.9435) -> (-25.2583, 31.7546) construction
  line L311 (-25.2261, 31.6978) -> (-25.196, 31.6399) construction
  spline S98 degree 4 poles (-25.2583, 31.7546) (-25.2261, 31.6978) (-25.196, 31.6399) (-25.1687, 31.5802) (-25.1538, 31.5163) knots 1 1 1 1 1 2 2 2 2 2
  line L312 (-25.2583, 31.7546) -> (-25.2261, 31.6978) construction
  line L313 (-25.196, 31.6399) -> (-25.1687, 31.5802) construction
  line L314 (-25.1687, 31.5802) -> (-25.1538, 31.5163) construction
  arc A54 (-25.1538, 31.5163) -> (-25.6736, 31.0943) centre (0, 0) ccw
  arc A55 (-25.6736, 31.0943) -> (-26.1864, 30.6637) centre (0, 0) ccw
  spline S99 degree 4 poles (-26.4006, 30.8115) (-26.3509, 30.7691) (-26.2997, 30.7285) (-26.2463, 30.6905) (-26.1864, 30.6637) knots 1 1 1 1 1 2 2 2 2 2
  line L315 (-26.4006, 30.8115) -> (-26.3509, 30.7691) construction
  line L316 (-26.3509, 30.7691) -> (-26.2997, 30.7285) construction
  line L317 (-26.2997, 30.7285) -> (-26.2463, 30.6905) construction
  line L318 (-26.2463, 30.6905) -> (-26.1864, 30.6637) construction
  line L319 (-31.5286, 29.5036) -> (-30.3317, 28.9212) construction
  spline S100 degree 2 poles (-31.5286, 29.5036) (-30.3317, 28.9212) (-29.2099, 28.1624) knots 1 1 1 2 2 2
  line L320 (-30.3317, 28.9212) -> (-29.2099, 28.1624) construction
  spline S101 degree 2 poles (-29.5036, 31.5286) (-28.9212, 30.3317) (-28.1624, 29.2099) knots 1 1 1 2 2 2
  line L321 (-29.5036, 31.5286) -> (-28.9212, 30.3317) construction
  line L322 (-28.9212, 30.3317) -> (-28.1624, 29.2099) construction
  line L323 (-28.125, 29.1564) -> (-28.0894, 29.1016) construction
  spline S102 degree 4 poles (-28.1624, 29.2099) (-28.125, 29.1564) (-28.0894, 29.1016) (-28.0566, 29.0447) (-28.0357, 28.9825) knots 1 1 1 1 1 2 2 2 2 2
  line L324 (-28.1624, 29.2099) -> (-28.125, 29.1564) construction
  line L325 (-28.0894, 29.1016) -> (-28.0566, 29.0447) construction
  line L326 (-28.0566, 29.0447) -> (-28.0357, 28.9825) construction
  arc A56 (-28.0357, 28.9825) -> (-28.5131, 28.5131) centre (0, 0) ccw
  arc A57 (-28.5131, 28.5131) -> (-28.9825, 28.0357) centre (0, 0) ccw
  spline S103 degree 4 poles (-29.2099, 28.1624) (-29.1564, 28.125) (-29.1016, 28.0894) (-29.0447, 28.0566) (-28.9825, 28.0357) knots 1 1 1 1 1 2 2 2 2 2
  line L327 (-29.2099, 28.1624) -> (-29.1564, 28.125) construction
  line L328 (-29.1564, 28.125) -> (-29.1016, 28.0894) construction
  line L329 (-29.1016, 28.0894) -> (-29.0447, 28.0566) construction
  line L330 (-29.0447, 28.0566) -> (-28.9825, 28.0357) construction
  line L331 (-34.1903, 26.373) -> (-32.9435, 25.907) construction
  spline S104 degree 2 poles (-34.1903, 26.373) (-32.9435, 25.907) (-31.7546, 25.2583) knots 1 1 1 2 2 2
  line L332 (-32.9435, 25.907) -> (-31.7546, 25.2583) construction
  spline S105 degree 2 poles (-32.367, 28.5813) (-31.6735, 27.4452) (-30.8115, 26.4006) knots 1 1 1 2 2 2
  line L333 (-32.367, 28.5813) -> (-31.6735, 27.4452) construction
  line L334 (-31.6735, 27.4452) -> (-30.8115, 26.4006) construction
  line L335 (-30.7691, 26.3509) -> (-30.7285, 26.2997) construction
  spline S106 degree 4 poles (-30.8115, 26.4006) (-30.7691, 26.3509) (-30.7285, 26.2997) (-30.6905, 26.2463) (-30.6637, 26.1864) knots 1 1 1 1 1 2 2 2 2 2
  line L336 (-30.8115, 26.4006) -> (-30.7691, 26.3509) construction
  line L337 (-30.7285, 26.2997) -> (-30.6905, 26.2463) construction
  line L338 (-30.6905, 26.2463) -> (-30.6637, 26.1864) construction
  arc A58 (-30.6637, 26.1864) -> (-31.0943, 25.6736) centre (0, 0) ccw
  arc A59 (-31.0943, 25.6736) -> (-31.5163, 25.1538) centre (0, 0) ccw
  spline S107 degree 4 poles (-31.7546, 25.2583) (-31.6978, 25.2261) (-31.6399, 25.196) (-31.5802, 25.1687) (-31.5163, 25.1538) knots 1 1 1 1 1 2 2 2 2 2
  line L339 (-31.7546, 25.2583) -> (-31.6978, 25.2261) construction
  line L340 (-31.6978, 25.2261) -> (-31.6399, 25.196) construction
  line L341 (-31.6399, 25.196) -> (-31.5802, 25.1687) construction
  line L342 (-31.5802, 25.1687) -> (-31.5163, 25.1538) construction
  line L343 (-36.5424, 23.0036) -> (-35.2569, 22.6583) construction
  spline S108 degree 2 poles (-36.5424, 23.0036) (-35.2569, 22.6583) (-34.0118, 22.1255) knots 1 1 1 2 2 2
  line L344 (-35.2569, 22.6583) -> (-34.0118, 22.1255) construction
  spline S109 degree 2 poles (-34.9372, 25.3752) (-34.1389, 24.3102) (-33.1815, 23.3522) knots 1 1 1 2 2 2
  line L345 (-34.9372, 25.3752) -> (-34.1389, 24.3102) construction
  line L346 (-34.1389, 24.3102) -> (-33.1815, 23.3522) construction
  line L347 (-33.1346, 23.3068) -> (-33.0893, 23.2597) construction
  spline S110 degree 4 poles (-33.1815, 23.3522) (-33.1346, 23.3068) (-33.0893, 23.2597) (-33.0464, 23.2101) (-33.014, 23.153) knots 1 1 1 1 1 2 2 2 2 2
  line L348 (-33.1815, 23.3522) -> (-33.1346, 23.3068) construction
  line L349 (-33.0893, 23.2597) -> (-33.0464, 23.2101) construction
  line L350 (-33.0464, 23.2101) -> (-33.014, 23.153) construction
  arc A60 (-33.014, 23.153) -> (-33.3939, 22.6017) centre (0, 0) ccw
  arc A61 (-33.3939, 22.6017) -> (-33.7646, 22.0441) centre (0, 0) ccw
  spline S111 degree 4 poles (-34.0118, 22.1255) (-33.9521, 22.0988) (-33.8916, 22.0743) (-33.8296, 22.0529) (-33.7646, 22.0441) knots 1 1 1 1 1 2 2 2 2 2
  line L351 (-34.0118, 22.1255) -> (-33.9521, 22.0988) construction
  line L352 (-33.9521, 22.0988) -> (-33.8916, 22.0743) construction
  line L353 (-33.8916, 22.0743) -> (-33.8296, 22.0529) construction
  line L354 (-33.8296, 22.0529) -> (-33.7646, 22.0441) construction
  line L355 (-38.5636, 19.4258) -> (-37.2511, 19.2043) construction
  spline S112 degree 2 poles (-38.5636, 19.4258) (-37.2511, 19.2043) (-35.9609, 18.7923) knots 1 1 1 2 2 2
  line L356 (-37.2511, 19.2043) -> (-35.9609, 18.7923) construction
  spline S113 degree 2 poles (-37.1911, 21.9393) (-36.2951, 20.955) (-35.251, 20.0924) knots 1 1 1 2 2 2
  line L357 (-37.1911, 21.9393) -> (-36.2951, 20.955) construction
  line L358 (-36.2951, 20.955) -> (-35.251, 20.0924) construction
  line L359 (-35.2, 20.0516) -> (-35.1505, 20.009) construction
  spline S114 degree 4 poles (-35.251, 20.0924) (-35.2, 20.0516) (-35.1505, 20.009) (-35.103, 19.9637) (-35.0654, 19.91) knots 1 1 1 1 1 2 2 2 2 2
  line L360 (-35.251, 20.0924) -> (-35.2, 20.0516) construction
  line L361 (-35.1505, 20.009) -> (-35.103, 19.9637) construction
  line L362 (-35.103, 19.9637) -> (-35.0654, 19.91) construction
  arc A62 (-35.0654, 19.91) -> (-35.3911, 19.325) centre (0, 0) ccw
  arc A63 (-35.3911, 19.325) -> (-35.7071, 18.7347) centre (0, 0) ccw
  spline S115 degree 4 poles (-35.9609, 18.7923) (-35.899, 18.7714) (-35.8364, 18.7528) (-35.7727, 18.7373) (-35.7071, 18.7347) knots 1 1 1 1 1 2 2 2 2 2
  line L363 (-35.9609, 18.7923) -> (-35.899, 18.7714) construction
  line L364 (-35.899, 18.7714) -> (-35.8364, 18.7528) construction
  line L365 (-35.8364, 18.7528) -> (-35.7727, 18.7373) construction
  line L366 (-35.7727, 18.7373) -> (-35.7071, 18.7347) construction
  line L367 (-40.2355, 15.6722) -> (-38.9079, 15.5764) construction
  spline S116 degree 2 poles (-40.2355, 15.6722) (-38.9079, 15.5764) (-37.5844, 15.2889) knots 1 1 1 2 2 2
  line L368 (-38.9079, 15.5764) -> (-37.5844, 15.2889) construction
  spline S117 degree 2 poles (-39.1082, 18.3048) (-38.1227, 17.41) (-37.0013, 16.6506) knots 1 1 1 2 2 2
  line L369 (-39.1082, 18.3048) -> (-38.1227, 17.41) construction
  line L370 (-38.1227, 17.41) -> (-37.0013, 16.6506) construction
  line L371 (-36.9466, 16.6148) -> (-36.8933, 16.5772) construction
  spline S118 degree 4 poles (-37.0013, 16.6506) (-36.9466, 16.6148) (-36.8933, 16.5772) (-36.8417, 16.5366) (-36.7992, 16.4867) knots 1 1 1 1 1 2 2 2 2 2
  line L372 (-37.0013, 16.6506) -> (-36.9466, 16.6148) construction
  line L373 (-36.8933, 16.5772) -> (-36.8417, 16.5366) construction
  line L374 (-36.8417, 16.5366) -> (-36.7992, 16.4867) construction
  arc A64 (-36.7992, 16.4867) -> (-37.0678, 15.8734) centre (0, 0) ccw
  arc A65 (-37.0678, 15.8734) -> (-37.3263, 15.2557) centre (0, 0) ccw
  spline S119 degree 4 poles (-37.5844, 15.2889) (-37.5208, 15.274) (-37.4567, 15.2614) (-37.3918, 15.252) (-37.3263, 15.2557) knots 1 1 1 1 1 2 2 2 2 2
  line L375 (-37.5844, 15.2889) -> (-37.5208, 15.274) construction
  line L376 (-37.5208, 15.274) -> (-37.4567, 15.2614) construction
  line L377 (-37.4567, 15.2614) -> (-37.3918, 15.252) construction
  line L378 (-37.3918, 15.252) -> (-37.3263, 15.2557) construction
  line L379 (-41.543, 11.7766) -> (-40.2124, 11.8074) construction
  spline S120 degree 2 poles (-41.543, 11.7766) (-40.2124, 11.8074) (-38.8675, 11.647) knots 1 1 1 2 2 2
  line L380 (-40.2124, 11.8074) -> (-38.8675, 11.647) construction
  spline S121 degree 2 poles (-40.6711, 14.5044) (-39.605, 13.7074) (-38.4165, 13.058) knots 1 1 1 2 2 2
  line L381 (-40.6711, 14.5044) -> (-39.605, 13.7074) construction
  line L382 (-39.605, 13.7074) -> (-38.4165, 13.058) construction
  line L383 (-38.3587, 13.0276) -> (-38.302, 12.9952) construction
  spline S122 degree 4 poles (-38.4165, 13.058) (-38.3587, 13.0276) (-38.302, 12.9952) (-38.2468, 12.9597) (-38.1997, 12.914) knots 1 1 1 1 1 2 2 2 2 2
  line L384 (-38.4165, 13.058) -> (-38.3587, 13.0276) construction
  line L385 (-38.302, 12.9952) -> (-38.2468, 12.9597) construction
  line L386 (-38.2468, 12.9597) -> (-38.1997, 12.914) construction
  arc A66 (-38.1997, 12.914) -> (-38.4088, 12.278) centre (0, 0) ccw
  arc A67 (-38.4088, 12.278) -> (-38.6074, 11.6385) centre (0, 0) ccw
  spline S123 degree 4 poles (-38.8675, 11.647) (-38.8028, 11.6382) (-38.7378, 11.6318) (-38.6723, 11.6287) (-38.6074, 11.6385) knots 1 1 1 1 1 2 2 2 2 2
  line L387 (-38.8675, 11.647) -> (-38.8028, 11.6382) construction
  line L388 (-38.8028, 11.6382) -> (-38.7378, 11.6318) construction
  line L389 (-38.7378, 11.6318) -> (-38.6723, 11.6287) construction
  line L390 (-38.6723, 11.6287) -> (-38.6074, 11.6385) construction
  line L391 (-42.4744, 7.7743) -> (-41.1526, 7.9315) construction
  spline S124 degree 2 poles (-42.4744, 7.7743) (-41.1526, 7.9315) (-39.7986, 7.8997) knots 1 1 1 2 2 2
  line L392 (-41.1526, 7.9315) -> (-39.7986, 7.8997) construction
  spline S125 degree 2 poles (-41.8656, 10.5727) (-40.7286, 9.8807) (-39.4838, 9.3471) knots 1 1 1 2 2 2
  line L393 (-41.8656, 10.5727) -> (-40.7286, 9.8807) construction
  line L394 (-40.7286, 9.8807) -> (-39.4838, 9.3471) construction
  line L395 (-39.4233, 9.3224) -> (-39.3638, 9.2955) construction
  spline S126 degree 4 poles (-39.4838, 9.3471) (-39.4233, 9.3224) (-39.3638, 9.2955) (-39.3055, 9.2654) (-39.2543, 9.2244) knots 1 1 1 1 1 2 2 2 2 2
  line L396 (-39.4838, 9.3471) -> (-39.4233, 9.3224) construction
  line L397 (-39.3638, 9.2955) -> (-39.3055, 9.2654) construction
  line L398 (-39.3055, 9.2654) -> (-39.2543, 9.2244) construction
  arc A68 (-39.2543, 9.2244) -> (-39.402, 8.5714) centre (0, 0) ccw
  arc A69 (-39.402, 8.5714) -> (-39.5389, 7.916) centre (0, 0) ccw
  spline S127 degree 4 poles (-39.7986, 7.8997) (-39.7334, 7.8971) (-39.6681, 7.8968) (-39.6025, 7.9) (-39.5389, 7.916) knots 1 1 1 1 1 2 2 2 2 2
  line L399 (-39.7986, 7.8997) -> (-39.7334, 7.8971) construction
  line L400 (-39.7334, 7.8971) -> (-39.6681, 7.8968) construction
  line L401 (-39.6681, 7.8968) -> (-39.6025, 7.9) construction
  line L402 (-39.6025, 7.9) -> (-39.5389, 7.916) construction
  line L403 (-43.021, 3.7017) -> (-41.7202, 3.9838) construction
  spline S128 degree 2 poles (-43.021, 3.7017) (-41.7202, 3.9838) (-40.3693, 4.0808) knots 1 1 1 2 2 2
  line L404 (-41.7202, 3.9838) -> (-40.3693, 4.0808) construction
  spline S129 degree 2 poles (-42.6811, 6.5452) (-41.4834, 5.9644) (-40.1935, 5.5517) knots 1 1 1 2 2 2
  line L405 (-42.6811, 6.5452) -> (-41.4834, 5.9644) construction
  line L406 (-41.4834, 5.9644) -> (-40.1935, 5.5517) construction
  line L407 (-40.131, 5.5328) -> (-40.0692, 5.5116) construction
  spline S130 degree 4 poles (-40.1935, 5.5517) (-40.131, 5.5328) (-40.0692, 5.5116) (-40.0083, 5.4872) (-39.9534, 5.4513) knots 1 1 1 1 1 2 2 2 2 2
  line L408 (-40.1935, 5.5517) -> (-40.131, 5.5328) construction
  line L409 (-40.0692, 5.5116) -> (-40.0083, 5.4872) construction
  line L410 (-40.0083, 5.4872) -> (-39.9534, 5.4513) construction
  arc A70 (-39.9534, 5.4513) -> (-40.0384, 4.7872) centre (0, 0) ccw
  arc A71 (-40.0384, 4.7872) -> (-40.1123, 4.1217) centre (0, 0) ccw
  spline S131 degree 4 poles (-40.3693, 4.0808) (-40.3041, 4.0844) (-40.2391, 4.0904) (-40.1742, 4.0997) (-40.1123, 4.1217) knots 1 1 1 1 1 2 2 2 2 2
  line L411 (-40.3693, 4.0808) -> (-40.3041, 4.0844) construction
  line L412 (-40.3041, 4.0844) -> (-40.2391, 4.0904) construction
  line L413 (-40.2391, 4.0904) -> (-40.1742, 4.0997) construction
  line L414 (-40.1742, 4.0997) -> (-40.1123, 4.1217) construction
  line L415 (-43.1781, -0.4045) -> (-41.91, 0) construction
  spline S132 degree 2 poles (-43.1781, -0.4045) (-41.91, 0) (-40.5744, 0.225) knots 1 1 1 2 2 2
  line L416 (-41.91, 0) -> (-40.5744, 0.225) construction
  spline S133 degree 2 poles (-43.11, 2.4585) (-41.8625, 1.9942) (-40.5392, 1.7059) knots 1 1 1 2 2 2
  line L417 (-43.11, 2.4585) -> (-41.8625, 1.9942) construction
  line L418 (-41.8625, 1.9942) -> (-40.5392, 1.7059) construction
  line L419 (-40.4752, 1.693) -> (-40.4117, 1.6779) construction
  spline S134 degree 4 poles (-40.5392, 1.7059) (-40.4752, 1.693) (-40.4117, 1.6779) (-40.3487, 1.6594) (-40.2906, 1.6288) knots 1 1 1 1 1 2 2 2 2 2